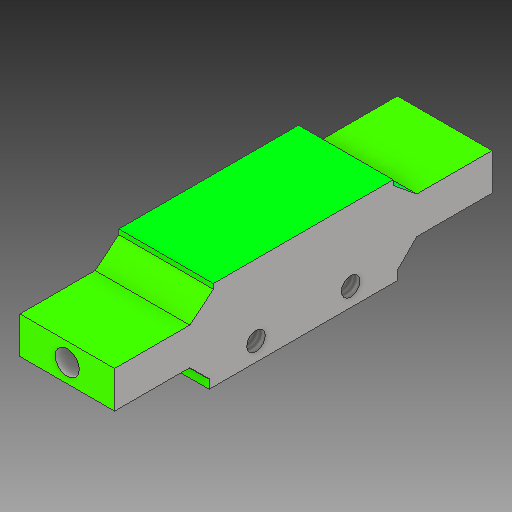
# Autodesk Inventor part: SliderSlider
Saved by Autodesk Inventor 2019 (Build 230136000, 136)
## iProperties
Created: 2019-10-06
Part Number: SliderSlider
Material: Generic
Document SubType Name: Modeling
Designer: james
Density: 1 g/cm^3
Appearance: Default
Author: james
Autodesk Inventor part; units mm, degrees
ref_plane "YZ Plane" through (0, 0, 0) normal (1, 0, 0) x (0, 1, 0)
ref_plane "XZ Plane" through (0, 0, 0) normal (0, 1, 0) x (-1, 0, 0)
ref_plane "XY Plane" through (0, 0, 0) normal (0, 0, 1) x (1, 0, 0)
sketch "Sketch1" plane through (0, 0, 0) normal (0, 0, 1) x (1, 0, 0)
  line L0 (-42.4234, 22.9681) -> (-17.0234, 22.9681)
  line L1 (-17.0234, 22.9681) -> (-17.0234, -2.4319)
  line L2 (-17.0234, -2.4319) -> (-42.4234, -2.4319)
  line L3 (-42.4234, -2.4319) -> (-42.4234, 22.9681)
  point P0 (0, 0)
  dimension "d0" = 25.4
  dimension "d1" = 25.4
  constraints: 8 end point, 2 parallel, 1 horizontal, 1 perpendicular
  measures "d0" distance of L1.end L2.end
  measures "d1" distance of L0.end L1.end
extrude "Extrusion1" add sketch "Sketch1" along normal blind 50.8
sketch "Sketch2" plane through (-17.0234, -2.4319, 0) normal (1, 0, 0) x (0, 0, -1)
  line L0 (-50.8, 22.86) -> (-50.8, 2.54)
  line L1 (-50.8, 2.54) -> (-55.88, 7.62)
  line L2 (-55.88, 7.62) -> (-76.2, 7.62)
  line L3 (-76.2, 7.62) -> (-76.2, 17.78)
  line L4 (-76.2, 17.78) -> (-55.88, 17.78)
  line L5 (-55.88, 17.78) -> (-50.8, 22.86)
  line L6 (-50.8, 0) -> (-50.8, 25.4) projected
  line L7 (0, 0) -> (-50.8, 0) projected
  point P0 (0, 2.4319)
  dimension "d4" = 25.4
  dimension "d5" = 20.32
  dimension "d6" = 5.08
  dimension "d7" = 5.08
  dimension "d8" = 5.08
  dimension "d9" = 5.08
  dimension "d10" = 0
  dimension "d11" = 2.54
  constraints: 12 end point, 3 perpendicular, 1 vertical
  measures "d4" distance between parallel lines of L0 L3
  measures "d5" distance of L0.start L0.end
  measures "d6" distance from line of L0.start L4
  measures "d7" horizontal distance of L0.end L1.end
  measures "d8" horizontal distance of L0.start L4.end
  measures "d9" horizontal distance of L0.end L1.end
  measures "d10" distance between parallel lines of L6 L0
  measures "d11" distance from line of L0.end L7
extrude "Extrusion2" add sketch "Sketch2" against normal blind 25.4
sketch "Sketch3" plane through (-17.0234, -2.4319, 0) normal (1, 0, 0) x (0, 0, -1)
  line L0 (0, 20.4965) -> (0, 2.54)
  line L1 (0, 2.54) -> (5.08, 7.62)
  line L2 (5.08, 7.62) -> (25.4, 7.62)
  line L3 (25.4, 7.62) -> (25.4, 17.78)
  line L4 (25.4, 17.78) -> (5.08, 17.78)
  line L5 (5.08, 17.78) -> (0, 22.86)
  line L6 (0, 22.86) -> (0, 20.4965)
  line L7 (-55.88, 7.62) -> (-76.2, 7.62) projected
  line L8 (-76.2, 17.78) -> (-55.88, 17.78) projected
  line L9 (0, 25.4) -> (0, 0) projected
  line L10 (0, 0) -> (-50.8, 0) projected
  point P0 (0, 2.4319)
  dimension "d14" = 20.32
  dimension "d15" = 5.08
  dimension "d16" = 5.08
  dimension "d17" = 5.08
  dimension "d18" = 5.08
  dimension "d19" = 25.4
  dimension "d20" = 10.16
  dimension "d21" = 0
  dimension "d22" = 2.54
  dimension "d23" = 10.16
  constraints: 14 end point, 3 perpendicular, 1 collinear, 1 point on line, 1 vertical
  measures "d14" distance of L0.end L5.end
  measures "d15" distance from line of L4 L5.end
  measures "d16" distance from line of L0.end L2
  measures "d17" distance from line of L0 L1.end
  measures "d18" horizontal distance of L5.end L4.end
  measures "d19" distance between parallel lines of L0 L3
  measures "d20" distance between parallel lines of L7 L8
  measures "d21" distance between parallel lines of L9 L0
  measures "d22" distance from line of L10 L0.end
  measures "d23" distance of L2.end L3.end
extrude "Extrusion3" add sketch "Sketch3" against normal blind 25.4
sketch "Sketch4" plane through (-17.0234, 5.1881, 76.2) normal (0, 0, 1) x (1, 0, 0)
  line L0 (0, 10.16) -> (-25.4, 10.16) projected
  line L1 (-25.4, 0) -> (-25.4, 10.16) projected
  point P0 (17.0234, -5.1881)
  point P1 (-12.7, 5.08)
  dimension "d26" = 5.08
  dimension "d27" = 12.7
  measures "d26" distance from line of point (-12.7, 5.08) L0
  measures "d27" distance from line of L1 point (-12.7, 5.08)
hole "Hole1" at (-29.7234, 10.2681, 76.2) direction (0, 0, -1) diameter 6.477 end through all
sketch "Sketch5" plane through (-17.0234, 22.9681, 50.8) normal (1, 0, 0) x (0, 0, -1)
  line L0 (50.8, -25.4) -> (0, -25.4) projected
  point P0 (50.8, -22.9681)
  point P1 (12.7, -20.32)
  point P2 (38.1, -20.32)
  dimension "d35" = 5.08
  dimension "d36" = 5.08
  dimension "d37" = 12.7
  dimension "d38" = 12.7
  measures "d35" distance from line of L0 point (38.1, -20.32)
  measures "d36" distance from line of L0 point (12.7, -20.32)
  measures "d37" horizontal distance of L0.end point (12.7, -20.32)
  measures "d38" horizontal distance of L0.start point (38.1, -20.32)
hole "Hole2" at (-17.0234, 2.6481, 38.1) at (-17.0234, 2.6481, 12.7) direction (-1, 0, 0) diameter 4.9784 end through all thread size "1/4-20 UNC" class "2B" standard "ANSI Unified Screw Threads"
sketch "Sketch7" plane through (-17.0234, 22.9681, 50.8) normal (1, 0, 0) x (0, 0, -1)
  line L0 (-29.4216, -5.046) -> (-25.273, -5.046)
  line L1 (-25.273, -5.046) -> (-25.273, -20.1383)
  line L2 (-25.273, -20.1383) -> (-29.4216, -20.1383)
  line L3 (-29.4216, -20.1383) -> (-29.4216, -5.046)
  line L4 (-25.4, -17.78) -> (-25.4, -7.62) projected
  point P0 (50.8, -22.9681)
  dimension "d62" = 0.127
  constraints: 8 end point, 2 parallel, 1 horizontal, 1 perpendicular
  measures "d62" distance between parallel lines of L4 L1
extrude "Extrusion4" cut sketch "Sketch7" against normal blind 50.8
sketch "Sketch8" plane through (-17.0234, -2.4319, 50.8) normal (1, 0, 0) x (0, 0, -1)
  line L0 (-27.9283, 21.8935) -> (-5.0883, 21.8935)
  line L1 (-5.0883, 21.8935) -> (-5.0883, 17.653)
  line L2 (-5.0883, 17.653) -> (-27.9283, 17.653)
  line L3 (-27.9283, 17.653) -> (-27.9283, 21.8935)
  line L4 (-25.273, 17.78) -> (-5.08, 17.78) projected
  line L5 (-26.1368, 7.747) -> (-5.0807, 7.747)
  line L6 (-5.0807, 7.747) -> (-5.0807, 5.4826)
  line L7 (-5.0807, 5.4826) -> (-26.1368, 5.4826)
  line L8 (-26.1368, 5.4826) -> (-26.1368, 7.747)
  line L9 (-5.08, 7.62) -> (-25.273, 7.62) projected
  point P0 (50.8, 2.4319)
  dimension "d65" = 0.127
  dimension "d66" = 0.127
  constraints: 16 end point, 4 parallel, 2 horizontal, 2 perpendicular
  measures "d65" distance between parallel lines of L2 L4
  measures "d66" distance between parallel lines of L9 L5
extrude "Extrusion5" cut sketch "Sketch8" against normal blind 50.8
sketch "Sketch9" plane through (-42.4234, 22.9681, 0) normal (-1, 0, 0) x (0, 0, 1)
  line L0 (-28.1622, -4.7577) -> (-5.0787, -4.7577)
  line L1 (-5.0787, -4.7577) -> (-5.0787, -7.747)
  line L2 (-5.0787, -7.747) -> (-28.1622, -7.747)
  line L3 (-28.1622, -7.747) -> (-28.1622, -4.7577)
  line L4 (-27.0984, -17.653) -> (-5.0787, -17.653)
  line L5 (-5.0787, -17.653) -> (-5.0787, -20.2143)
  line L6 (-5.0787, -20.2143) -> (-27.0984, -20.2143)
  line L7 (-27.0984, -20.2143) -> (-27.0984, -17.653)
  line L8 (-29.1947, -5.6651) -> (-25.273, -5.6651)
  line L9 (-25.273, -5.6651) -> (-25.273, -18.8063)
  line L10 (-25.273, -18.8063) -> (-29.1947, -18.8063)
  line L11 (-29.1947, -18.8063) -> (-29.1947, -5.6651)
  line L12 (-25.4, -7.62) -> (-25.4, -17.78) projected
  line L13 (-5.08, -7.62) -> (-25.4, -7.62) projected
  line L14 (-25.4, -17.78) -> (-5.08, -17.78) projected
  point P0 (0, -22.9681)
  dimension "d69" = 0.127
  dimension "d70" = 0.127
  dimension "d71" = 0.127
  constraints: 24 end point, 6 parallel, 3 horizontal, 3 perpendicular, 1 point on line
  measures "d69" distance between parallel lines of L9 L12
  measures "d70" distance between parallel lines of L13 L2
  measures "d71" distance between parallel lines of L14 L4
extrude "Extrusion6" cut sketch "Sketch9" against normal blind 50.8
sketch "Sketch10" plane through (-42.4234, -2.4319, 0) normal (-1, 0, 0) x (0, 0, 1)
  line L0 (-2.7564, 0.127) -> (53.3126, 0.127)
  line L1 (53.3126, 0.127) -> (53.3126, -2.1248)
  line L2 (53.3126, -2.1248) -> (-2.7564, -2.1248)
  line L3 (-2.7564, -2.1248) -> (-2.7564, 0.127)
  line L4 (50.673, -3.7518) -> (52.4991, -3.7518)
  line L5 (52.4991, -3.7518) -> (52.4991, 2.4319)
  line L6 (52.4991, 2.4319) -> (50.673, 2.4319)
  line L7 (50.673, 2.4319) -> (50.673, -3.7518)
  line L8 (0.127, -3.5953) -> (-2.3183, -3.5953)
  line L9 (-2.3183, -3.5953) -> (-2.3183, 2.4319)
  line L10 (-2.3183, 2.4319) -> (0.127, 2.4319)
  line L11 (0.127, 2.4319) -> (0.127, -3.5953)
  line L12 (0, 0) -> (0, 2.54) projected
  line L13 (0, 0) -> (50.8, 0) projected
  line L14 (50.8, 2.54) -> (50.8, 0) projected
  point P0 (0, 2.4319)
  dimension "d74" = 0.127
  dimension "d75" = 0.127
  dimension "d76" = 0.127
  constraints: 24 end point, 6 parallel, 3 horizontal, 3 perpendicular, 1 point on line
  measures "d74" distance between parallel lines of L12 L11
  measures "d75" distance between parallel lines of L13 L0
  measures "d76" distance between parallel lines of L14 L7
extrude "Extrusion7" cut sketch "Sketch10" against normal blind 50.8
sketch "Sketch11" plane through (-42.4234, 22.9681, 0) normal (-1, 0, 0) x (0, 0, 1)
  line L0 (-3.471, 3.7894) -> (53.579, 3.7894)
  line L1 (53.579, 3.7894) -> (53.579, -1.27)
  line L2 (53.579, -1.27) -> (-3.471, -1.27)
  line L3 (-3.471, -1.27) -> (-3.471, 3.7894)
  line L4 (49.53, 5.7803) -> (53.579, 5.7803)
  line L5 (53.579, 5.7803) -> (53.579, -2.5925)
  line L6 (53.579, -2.5925) -> (49.53, -2.5925)
  line L7 (49.53, -2.5925) -> (49.53, 5.7803)
  line L8 (1.27, 6.2042) -> (-3.2289, 6.2042)
  line L9 (-3.2289, 6.2042) -> (-3.2289, -2.5925)
  line L10 (-3.2289, -2.5925) -> (1.27, -2.5925)
  line L11 (1.27, -2.5925) -> (1.27, 6.2042)
  line L12 (0, -2.54) -> (0, 0) projected
  line L13 (0, 0) -> (50.8, 0) projected
  line L14 (50.8, 0) -> (50.8, -2.54) projected
  point P0 (0, -22.9681)
  dimension "d79" = 1.27
  dimension "d80" = 1.27
  dimension "d81" = 1.27
  constraints: 24 end point, 6 parallel, 3 horizontal, 3 perpendicular, 2 point on line
  measures "d79" distance between parallel lines of L12 L11
  measures "d80" distance between parallel lines of L13 L2
  measures "d81" distance between parallel lines of L14 L7
extrude "Extrusion8" cut sketch "Sketch11" against normal blind 50.8
sketch "Sketch13" plane through (-42.4234, 5.3151, 76.073) normal (-1, 0, 0) x (0, 0, 1)
  line L0 (-81.1517, 0) -> (-81.1517, -0.1283) projected
  line L1 (-81.1517, 0) -> (-81.1517, -0.1283)
  line L2 (-81.1517, -0.1283) -> (-76.073, -5.207)
  line L3 (-81.1517, -0.1283) -> (-76.073, -5.207) projected
  line L4 (-76.073, -5.3151) -> (-75.946, -5.3151) projected
  line L5 (-76.073, -5.3151) -> (-75.946, -5.3151)
  line L6 (-75.946, -5.3151) -> (-75.946, -5.2062)
  line L7 (-76.073, -5.3151) -> (-76.073, -5.207) projected
  line L8 (-76.073, -5.3151) -> (-76.073, -5.207)
  line L9 (-81.1517, 0) -> (-75.946, -5.2062)
  constraints: 13 end point, 3 collinear, 1 perpendicular
extrude "Extrusion9" cut sketch "Sketch13" against normal blind 50.8
sketch "Sketch14" plane through (-42.4234, 5.3151, 76.073) normal (-1, 0, 0) x (0, 0, 1)
  line L0 (-81.1517, 9.906) -> (-81.1517, 10.0343) projected
  line L1 (-81.1517, 9.906) -> (-81.1517, 10.0343)
  line L2 (-76.1255, 15.0605) -> (-74.803, 15.0605) projected
  line L3 (-81.1517, 10.0343) -> (-76.1255, 15.0605)
  line L4 (-81.1517, 10.0343) -> (-76.1255, 15.0605) projected
  line L5 (-76.1255, 15.0605) -> (-74.803, 15.0605)
  line L6 (-74.803, 15.0605) -> (-74.803, 16.383) projected
  line L7 (-74.803, 15.0605) -> (-81.1517, 9.906)
  point P0 (-76.073, -5.3151)
  constraints: 8 end point, 1 collinear, 1 vertical
extrude "Extrusion10" cut sketch "Sketch14" against normal blind 50.8
sketch "Sketch16" plane through (-42.4234, 5.3151, 76.073) normal (-1, 0, 0) x (0, 0, 1)
  line L0 (-26.543, 15.0605) -> (-26.543, 16.383) projected
  line L1 (-20.193, 10.033) -> (-25.2205, 15.0605) projected
  line L2 (-26.543, 15.0605) -> (-25.2205, 15.0605)
  line L3 (-20.1847, 9.906) -> (-20.1847, 10.033) projected
  line L4 (-25.2205, 15.0605) -> (-20.1847, 10.033)
  line L5 (-26.543, 15.0605) -> (-20.1847, 9.906)
  line L6 (0, 9.906) -> (-20.1847, 9.906) projected
  line L7 (-20.1847, 9.906) -> (-20.1847, 10.033)
  point P0 (-76.073, -5.3151)
  constraints: 8 end point, 1 horizontal, 1 point on line, 1 vertical
extrude "Extrusion11" cut sketch "Sketch16" against normal blind 50.8
sketch "Sketch18" plane through (-42.4234, 5.3151, 76.073) normal (-1, 0, 0) x (0, 0, 1)
  line L0 (-20.1923, 0) -> (-20.1923, -0.127) projected
  line L1 (-20.1923, 0) -> (-25.5398, -5.3151)
  line L2 (-25.5398, -5.3151) -> (-25.1146, -5.3151)
  line L3 (-25.1146, -5.3151) -> (-20.1923, -0.127)
  point P0 (-76.073, -5.3151)
  constraints: 6 end point, 1 perpendicular
extrude "Extrusion12" cut sketch "Sketch18" against normal blind 50.8
body "Solid1"
